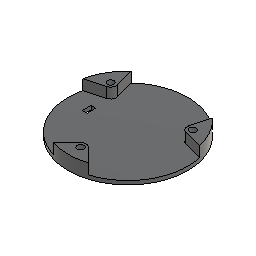
RGB_ChristmasLight_Base_Enclosure_Bottom_v1 (Autodesk Fusion 360 design; units mm, degrees)
Autodesk Fusion 360 part; units mm, degrees
(part 1 of 2)
sketch "Sketch1" plane through (0, 0, 0) normal (0, 0, 1) x (1, 0, 0)
  circle A0 centre (0, 0) radius 31.5
  circle A1 centre (0, 0) radius 30 construction
  circle A2 centre (0, 0) radius 25 construction
  circle A3 centre (0, -25) radius 1.75
  circle A4 centre (21.6506, 12.5) radius 1.75
  circle A5 centre (-21.6506, 12.5) radius 1.75
  line L0 (-30, 0) -> (-20.5, 0) construction
  line L1 (-20.5, 0) -> (-19.25, 0) construction
  line L2 (-19.25, 0) -> (-19.25, 2.25) construction
  line L3 (-19.25, 2.25) -> (-20.5, 2.25) construction
  line L4 (-20.5, 2.25) -> (-20.5, 0) construction
  line L5 (-19.25, 2.25) -> (-21.75, 2.25)
  line L6 (-21.75, 2.25) -> (-21.75, -2.25)
  line L7 (-21.75, -2.25) -> (-19.25, -2.25)
  line L8 (-19.25, -2.25) -> (-19.25, 2.25)
  dimension "d1_1" = 63
  dimension "d84" = 60
  dimension "d85" = -5
  dimension "d86" = 3.5
  dimension "d88" = 360
  dimension "d89" = 9.5
  dimension "d90" = 1.25
  dimension "d91" = 2.25
  dimension "d92" = 2.5
  dimension "d93" = 4.5
  constraint coincident A0.centre A1.centre
  constraint coincident A2 A3.centre
  constraint coincident A1 L0.start
  constraint horizontal L0
  constraint horizontal L1
  constraint vertical L2
  constraint horizontal L3
  constraint vertical L4
  constraint horizontal L5
  constraint vertical L6
  constraint horizontal L7
  constraint vertical L8
  measures "d1_1" diameter of A0
  measures "d84" diameter of A1
  measures "d86" diameter of A3
  measures "d89" distance of L0.start L0.end
  measures "d90" distance of L0.end L1.end
  measures "d91" distance of L0.end L3.end
  measures "d92" distance of L2.end L5.end
  measures "d93" distance of L2.end L7.end
extrude "Extrude1" add sketch "Sketch1" along normal blind 2 contours A0 | A3 | A4 | A5 | L5 L6 L7 L8
extrude "Extrude5" cut sketch "Sketch1" along normal blind 2 contours A3 | A4 | A5 | L5 L6 L7 L8
sketch "Sketch3" plane through (0, 0, 2) normal (0, 0, 1) x (-1, 0, 0)
  line L0 (19.25, 2.25) -> (21.75, 2.25)
  line L1 (21.75, 2.25) -> (21.75, -2.25)
  line L2 (21.75, -2.25) -> (19.25, -2.25)
  line L3 (19.25, -2.25) -> (19.25, 2.25)
  circle A0 centre (0, 25) radius 1.75
  circle A1 centre (21.6506, -12.5) radius 1.75
  circle A2 centre (-21.6506, -12.5) radius 1.75
  circle A3 centre (0, 0) radius 31.5
  arc A4 (2.1213, 22.8787) -> (0, 22) centre (0, 25) cw
  arc A5 (0, 22) -> (-2.1213, 22.8787) centre (0, 25) cw
  line L4 (-2.1213, 22.8787) -> (-9.3294, 30.0867)
  line L5 (2.1213, 22.8787) -> (9.3294, 30.0867)
  line L6 (-20.8742, -9.6022) -> (-30.7206, -6.9639)
  arc A6 (-20.8742, -9.6022) -> (-19.0526, -11) centre (-21.6506, -12.5) cw
  arc A7 (-19.0526, -11) -> (-18.7529, -13.2765) centre (-21.6506, -12.5) cw
  line L7 (-18.7529, -13.2765) -> (-21.3912, -23.1229)
  line L8 (18.7529, -13.2765) -> (21.3912, -23.1229)
  arc A8 (18.7529, -13.2765) -> (19.0526, -11) centre (21.6506, -12.5) cw
  arc A9 (19.0526, -11) -> (20.8742, -9.6022) centre (21.6506, -12.5) cw
  line L9 (20.8742, -9.6022) -> (30.7206, -6.9639)
  dimension "d108" = 360
extrude "Extrude6" add sketch "Sketch3" along normal blind 5.45 contours A3 A4 A5 L4 L5 | A3 L8 A8 A9 L9 | A3 L6 A6 A7 L7
sketch "Sketch4" plane through (0, 0, 0) normal (0, 0, -1) x (1, 0, 0)
  line L0 (-21.75, 2.25) -> (-19.25, 2.25)
  line L1 (-19.25, 2.25) -> (-19.25, -2.25)
  line L2 (-19.25, -2.25) -> (-21.75, -2.25)
  line L3 (-21.75, -2.25) -> (-21.75, 2.25)
  circle A0 centre (0, 25) radius 1.75
  circle A1 centre (-21.6506, -12.5) radius 1.75
  circle A2 centre (21.6506, -12.5) radius 1.75
  circle A3 centre (0, 0) radius 31.5
  spline S0 degree 3 poles (-1.0856, -16.0234) (-1.0936, -16.0234) (-1.2047, -15.8091) (-1.3357, -15.5472) knots 0 0 0 0 1 1 1 1
  spline S1 degree 3 poles (-1.3357, -15.5472) (-1.4666, -15.2852) (-1.5738, -15.0551) (-1.5738, -15.0312) knots 0 0 0 0 1 1 1 1
  spline S2 degree 3 poles (-1.5738, -15.0312) (-1.5738, -14.9916) (-1.1491, -15.0074) (-0.6729, -15.067) knots 0 0 0 0 1 1 1 1
  line L4 (-0.6729, -15.067) -> (-0.4626, -15.0908)
  line L5 (-0.4626, -15.0908) -> (-0.7721, -15.5551)
  spline S3 degree 3 poles (-0.7721, -15.5551) (-0.9388, -15.8131) (-1.0817, -16.0234) (-1.0856, -16.0234) knots 0 0 0 0 1 1 1 1
  spline S4 degree 3 poles (15.4005, 7.3843) (15.3728, 7.3684) (14.8806, 7.0787) (14.3012, 6.7413) knots -1 -1 -1 -1 0 0 0 0
  spline S5 degree 3 poles (14.7139, 8.682) (15.2219, 7.8049) (15.4323, 7.4041) (15.4005, 7.3843) knots -1 -1 -1 -1 0 0 0 0
  spline S6 degree 3 poles (13.948, 9.9838) (13.9639, 9.9679) (14.3091, 9.3805) (14.7139, 8.682) knots -1 -1 -1 -1 0 0 0 0
  spline S7 degree 3 poles (13.6583, 9.8608) (13.8011, 9.9441) (13.9321, 9.9997) (13.948, 9.9838) knots -1 -1 -1 -1 0 0 0 0
  line L6 (13.3963, 9.7099) -> (13.6583, 9.8608)
  line L7 (14.3726, 8.0272) -> (13.3963, 9.7099)
  line L8 (14.2496, 7.9518) -> (14.3726, 8.0272)
  spline S8 degree 3 poles (13.4876, 7.5113) (13.8369, 7.7137) (14.1782, 7.9121) (14.2496, 7.9518) knots -1 -1 -1 -1 0 0 0 0
  spline S9 degree 3 poles (12.7653, 7.0906) (12.8129, 7.1223) (13.1384, 7.3089) (13.4876, 7.5113) knots -1 -1 -1 -1 0 0 0 0
  spline S10 degree 3 poles (12.9439, 6.5786) (12.6819, 7.035) (12.6819, 7.039) (12.7653, 7.0906) knots -1 -1 -1 -1 0 0 0 0
  spline S11 degree 3 poles (13.2296, 6.1262) (13.2177, 6.1222) (13.0907, 6.3286) (12.9439, 6.5786) knots -1 -1 -1 -1 0 0 0 0
  spline S12 degree 3 poles (14.3012, 6.7413) (13.7218, 6.404) (13.2415, 6.1262) (13.2296, 6.1262) knots -1 -1 -1 -1 0 0 0 0
  spline S13 degree 3 poles (-13.8214, 4.5545) (-13.8293, 3.7092) (-14.2262, 2.8599) (-14.7104, 2.6535) knots -1 -1 -1 -1 0 0 0 0
  spline S14 degree 3 poles (-13.9325, 5.1618) (-13.8253, 4.9673) (-13.8174, 4.9236) (-13.8214, 4.5545) knots -1 -1 -1 -1 0 0 0 0
  spline S15 degree 3 poles (-14.7104, 5.6063) (-14.4286, 5.6817) (-14.127, 5.507) (-13.9325, 5.1618) knots -1 -1 -1 -1 0 0 0 0
  spline S16 degree 3 poles (-15.4843, 4.4156) (-15.2025, 5.2094) (-14.9921, 5.5308) (-14.7104, 5.6063) knots -1 -1 -1 -1 0 0 0 0
  spline S17 degree 3 poles (-15.8454, 4.0386) (-15.7383, 3.7886) (-15.6867, 3.8441) (-15.4843, 4.4156) knots -1 -1 -1 -1 0 0 0 0
  spline S18 degree 3 poles (-15.6827, 4.6538) (-15.8613, 4.4672) (-15.9248, 4.2291) (-15.8454, 4.0386) knots -1 -1 -1 -1 0 0 0 0
  spline S19 degree 3 poles (-15.5279, 4.8919) (-15.5438, 4.8363) (-15.6113, 4.7292) (-15.6827, 4.6538) knots -1 -1 -1 -1 0 0 0 0
  spline S20 degree 3 poles (-15.389, 5.4158) (-15.4525, 5.1816) (-15.516, 4.9474) (-15.5279, 4.8919) knots -1 -1 -1 -1 0 0 0 0
  line L9 (-15.2739, 5.8444) -> (-15.389, 5.4158)
  line L10 (-15.4366, 5.8206) -> (-15.2739, 5.8444)
  spline S21 degree 3 poles (-16.54, 4.4275) (-16.3415, 5.2848) (-15.9843, 5.7333) (-15.4366, 5.8206) knots -1 -1 -1 -1 0 0 0 0
  spline S22 degree 3 poles (-16.2145, 2.9115) (-16.5955, 3.1853) (-16.7066, 3.7013) (-16.54, 4.4275) knots -1 -1 -1 -1 0 0 0 0
  spline S23 degree 3 poles (-14.9088, 4.0465) (-15.3255, 2.8519) (-15.6946, 2.5305) (-16.2145, 2.9115) knots -1 -1 -1 -1 0 0 0 0
  spline S24 degree 3 poles (-14.6111, 4.4315) (-14.6985, 4.5466) (-14.762, 4.4633) (-14.9088, 4.0465) knots -1 -1 -1 -1 0 0 0 0
  spline S25 degree 3 poles (-14.762, 3.7171) (-14.5715, 3.864) (-14.4841, 4.2648) (-14.6111, 4.4315) knots -1 -1 -1 -1 0 0 0 0
  spline S26 degree 3 poles (-14.9882, 3.1853) (-14.889, 3.5425) (-14.8413, 3.6576) (-14.762, 3.7171) knots -1 -1 -1 -1 0 0 0 0
  spline S27 degree 3 poles (-15.1311, 2.6575) (-15.1191, 2.6972) (-15.0556, 2.9353) (-14.9882, 3.1853) knots -1 -1 -1 -1 0 0 0 0
  spline S28 degree 3 poles (-15.0001, 2.59) (-15.1271, 2.59) (-15.1469, 2.6019) (-15.1311, 2.6575) knots -1 -1 -1 -1 0 0 0 0
  spline S29 degree 3 poles (-14.7104, 2.6535) (-14.7858, 2.6218) (-14.9167, 2.594) (-15.0001, 2.59) knots -1 -1 -1 -1 0 0 0 0
  spline S30 degree 3 poles (16.7856, 3.1893) (16.7658, 3.1814) (16.2181, 3.0266) (15.5752, 2.848) knots -1 -1 -1 -1 0 0 0 0
  spline S31 degree 3 poles (15.9998, 6.1857) (16.0474, 6.1381) (16.8174, 3.2012) (16.7856, 3.1893) knots -1 -1 -1 -1 0 0 0 0
  spline S32 degree 3 poles (15.4244, 6.0269) (15.4482, 6.0508) (15.9839, 6.1976) (15.9998, 6.1857) knots -1 -1 -1 -1 0 0 0 0
  spline S33 degree 3 poles (15.6704, 5.0506) (15.5275, 5.5824) (15.4164, 6.019) (15.4244, 6.0269) knots -1 -1 -1 -1 0 0 0 0
  spline S34 degree 3 poles (15.9165, 4.0743) (15.9284, 4.0823) (15.8173, 4.5228) (15.6704, 5.0506) knots -1 -1 -1 -1 0 0 0 0
  spline S35 degree 3 poles (15.718, 3.9989) (15.8173, 4.0267) (15.9046, 4.0624) (15.9165, 4.0743) knots -1 -1 -1 -1 0 0 0 0
  line L11 (15.5355, 3.9434) -> (15.718, 3.9989)
  line L12 (15.4759, 4.1497) -> (15.5355, 3.9434)
  spline S36 degree 3 poles (15.2696, 4.8919) (15.3529, 4.5982) (15.4442, 4.2648) (15.4759, 4.1497) knots -1 -1 -1 -1 0 0 0 0
  spline S37 degree 3 poles (15.0949, 5.4594) (15.1108, 5.4435) (15.1902, 5.1856) (15.2696, 4.8919) knots -1 -1 -1 -1 0 0 0 0
  spline S38 degree 3 poles (14.6862, 5.3681) (14.7497, 5.4197) (15.0672, 5.4912) (15.0949, 5.4594) knots -1 -1 -1 -1 0 0 0 0
  spline S39 degree 3 poles (14.8568, 4.5942) (14.7457, 5.003) (14.6663, 5.3523) (14.6862, 5.3681) knots -1 -1 -1 -1 0 0 0 0
  spline S40 degree 3 poles (15.0434, 3.8322) (15.0513, 3.8441) (14.9679, 4.1854) (14.8568, 4.5942) knots -1 -1 -1 -1 0 0 0 0
  spline S41 degree 3 poles (14.8409, 3.7608) (14.9402, 3.7886) (15.0314, 3.8243) (15.0434, 3.8322) knots -1 -1 -1 -1 0 0 0 0
  spline S42 degree 3 poles (14.6385, 3.7529) (14.6504, 3.7132) (14.6981, 3.7171) (14.8409, 3.7608) knots -1 -1 -1 -1 0 0 0 0
  spline S43 degree 3 poles (14.3964, 4.6339) (14.5195, 4.1735) (14.6306, 3.7806) (14.6385, 3.7529) knots -1 -1 -1 -1 0 0 0 0
  spline S44 degree 3 poles (14.1424, 5.4991) (14.1583, 5.4832) (14.2734, 5.0903) (14.3964, 4.6339) knots -1 -1 -1 -1 0 0 0 0
  spline S45 degree 3 poles (13.5709, 5.3245) (13.567, 5.388) (14.0988, 5.5507) (14.1424, 5.4991) knots -1 -1 -1 -1 0 0 0 0
  spline S46 degree 3 poles (14.2655, 2.7765) (14.1147, 3.3044) (13.5749, 5.2689) (13.5709, 5.3245) knots -1 -1 -1 -1 0 0 0 0
  spline S47 degree 3 poles (14.3726, 2.5146) (14.3568, 2.5106) (14.3091, 2.6297) (14.2655, 2.7765) knots -1 -1 -1 -1 0 0 0 0
  spline S48 degree 3 poles (15.5752, 2.848) (14.9283, 2.6654) (14.3885, 2.5186) (14.3726, 2.5146) knots -1 -1 -1 -1 0 0 0 0
  spline S49 degree 3 poles (8.3917, 2.8242) (8.4513, 2.6337) (8.3838, 2.4313) (8.225, 2.2924) knots -1 -1 -1 -1 0 0 0 0
  spline S50 degree 3 poles (7.9353, 3.1774) (8.1893, 3.1575) (8.3243, 3.0504) (8.3917, 2.8242) knots -1 -1 -1 -1 0 0 0 0
  spline S51 degree 3 poles (7.5702, 3.0544) (7.7131, 3.1853) (7.7369, 3.1933) (7.9353, 3.1774) knots -1 -1 -1 -1 0 0 0 0
  spline S52 degree 3 poles (7.4154, 2.6892) (7.4154, 2.8996) (7.4273, 2.9234) (7.5702, 3.0544) knots -1 -1 -1 -1 0 0 0 0
  spline S53 degree 3 poles (7.5623, 2.3281) (7.4273, 2.4551) (7.4154, 2.4789) (7.4154, 2.6892) knots -1 -1 -1 -1 0 0 0 0
  spline S54 degree 3 poles (7.9075, 2.1931) (7.7409, 2.1931) (7.6893, 2.213) (7.5623, 2.3281) knots -1 -1 -1 -1 0 0 0 0
  spline S55 degree 3 poles (8.225, 2.2924) (8.1298, 2.2169) (8.0584, 2.1931) (7.9075, 2.1931) knots -1 -1 -1 -1 0 0 0 0
  spline S56 degree 3 poles (-8.2016, 3.0663) (-7.7016, 3.0663) (-7.5071, 2.4709) (-7.9079, 2.1574) knots -1 -1 -1 -1 0 0 0 0
  spline S57 degree 3 poles (-8.658, 2.7884) (-8.5628, 2.975) (-8.412, 3.0663) (-8.2016, 3.0663) knots -1 -1 -1 -1 0 0 0 0
  spline S58 degree 3 poles (-8.2016, 2.0741) (-8.5826, 2.0741) (-8.8287, 2.4551) (-8.658, 2.7884) knots -1 -1 -1 -1 0 0 0 0
  spline S59 degree 3 poles (-7.9079, 2.1574) (-7.9833, 2.0979) (-8.0706, 2.0741) (-8.2016, 2.0741) knots -1 -1 -1 -1 0 0 0 0
  spline S60 degree 3 poles (6.963, -0.1326) (7.0622, -0.3548) (7.0146, -0.5691) (6.836, -0.7199) knots -1 -1 -1 -1 0 0 0 0
  spline S61 degree 3 poles (6.0065, -0.327) (6.0065, 0.2167) (6.7447, 0.3635) (6.963, -0.1326) knots -1 -1 -1 -1 0 0 0 0
  spline S62 degree 3 poles (6.5383, -0.8231) (6.2089, -0.8231) (6.0065, -0.6366) (6.0065, -0.327) knots -1 -1 -1 -1 0 0 0 0
  spline S63 degree 3 poles (6.836, -0.7199) (6.7447, -0.7993) (6.6693, -0.8231) (6.5383, -0.8231) knots -1 -1 -1 -1 0 0 0 0
  spline S64 degree 3 poles (10.134, 0.7287) (10.134, 0.5818) (10.1102, 0.5342) (9.9792, 0.4032) knots -1 -1 -1 -1 0 0 0 0
  spline S65 degree 3 poles (9.3045, 1.1374) (9.6498, 1.4311) (10.134, 1.193) (10.134, 0.7287) knots -1 -1 -1 -1 0 0 0 0
  spline S66 degree 3 poles (9.2172, 0.4509) (9.0744, 0.7168) (9.1061, 0.9747) (9.3045, 1.1374) knots -1 -1 -1 -1 0 0 0 0
  spline S67 degree 3 poles (9.6617, 0.2484) (9.4673, 0.2484) (9.2807, 0.3358) (9.2172, 0.4509) knots -1 -1 -1 -1 0 0 0 0
  spline S68 degree 3 poles (9.9792, 0.4032) (9.8522, 0.2723) (9.8006, 0.2484) (9.6617, 0.2484) knots -1 -1 -1 -1 0 0 0 0
  spline S69 degree 3 poles (-5.9394, 0.4469) (-5.9394, 0.1849) (-6.0863, -0.0214) (-6.3165, -0.081) knots -1 -1 -1 -1 0 0 0 0
  spline S70 degree 3 poles (-6.3641, 0.9112) (-6.1299, 0.8795) (-5.9394, 0.6731) (-5.9394, 0.4469) knots -1 -1 -1 -1 0 0 0 0
  spline S71 degree 3 poles (-6.9475, 0.4866) (-6.8959, 0.7842) (-6.6697, 0.9509) (-6.3641, 0.9112) knots -1 -1 -1 -1 0 0 0 0
  spline S72 degree 3 poles (-6.3165, -0.081) (-6.6419, -0.1643) (-7.007, 0.1611) (-6.9475, 0.4866) knots -1 -1 -1 -1 0 0 0 0
  spline S73 degree 3 poles (8.5187, -10.4156) (6.2645, -12.2134) (3.6332, -13.2374) (0.8273, -13.4041) knots -1 -1 -1 -1 0 0 0 0
  spline S74 degree 3 poles (10.5071, -8.4233) (10.0705, -8.971) (9.0545, -9.987) (8.5187, -10.4156) knots -1 -1 -1 -1 0 0 0 0
  spline S75 degree 3 poles (13.3249, -2.0852) (12.9677, -4.3632) (11.9954, -6.558) (10.5071, -8.4233) knots -1 -1 -1 -1 0 0 0 0
  line L13 (13.3765, -1.7359) -> (13.3249, -2.0852)
  line L14 (11.9676, -1.7359) -> (13.3765, -1.7359)
  line L15 (11.7255, -2.1487) -> (11.9676, -1.7359)
  spline S76 degree 3 poles (11.4358, -2.5773) (11.4635, -2.5694) (11.5945, -2.3749) (11.7255, -2.1487) knots -1 -1 -1 -1 0 0 0 0
  spline S77 degree 3 poles (10.1856, -2.5932) (10.8444, -2.5932) (11.408, -2.5892) (11.4358, -2.5773) knots -1 -1 -1 -1 0 0 0 0
  line L16 (8.991, -2.5892) -> (10.1856, -2.5932)
  line L17 (8.9474, -2.7361) -> (8.991, -2.5892)
  spline S78 degree 3 poles (8.5187, -3.1686) (8.6854, -3.1051) (8.8997, -2.8869) (8.9474, -2.7361) knots -1 -1 -1 -1 0 0 0 0
  spline S79 degree 3 poles (7.979, -3.1488) (8.1298, -3.2123) (8.3798, -3.2202) (8.5187, -3.1686) knots -1 -1 -1 -1 0 0 0 0
  spline S80 degree 3 poles (7.5146, -2.4701) (7.5146, -2.7083) (7.7528, -3.0575) (7.979, -3.1488) knots -1 -1 -1 -1 0 0 0 0
  spline S81 degree 3 poles (7.717, -1.9939) (7.6139, -2.113) (7.5146, -2.3471) (7.5146, -2.4701) knots -1 -1 -1 -1 0 0 0 0
  spline S82 degree 3 poles (8.9275, -2.1884) (8.7291, -1.7002) (8.0663, -1.597) (7.717, -1.9939) knots -1 -1 -1 -1 0 0 0 0
  line L18 (9.0029, -2.3709) -> (8.9275, -2.1884)
  line L19 (11.3445, -2.3709) -> (9.0029, -2.3709)
  line L20 (11.5826, -1.9621) -> (11.3445, -2.3709)
  line L21 (11.8207, -1.5573) -> (11.5826, -1.9621)
  line L22 (12.6026, -1.5454) -> (11.8207, -1.5573)
  spline S83 degree 3 poles (13.4003, -1.4819) (13.3844, -1.5256) (13.2019, -1.5375) (12.6026, -1.5454) knots -1 -1 -1 -1 0 0 0 0
  spline S84 degree 3 poles (13.4479, -1.0295) (13.432, -1.2478) (13.4122, -1.4541) (13.4003, -1.4819) knots -1 -1 -1 -1 0 0 0 0
  spline S85 degree 3 poles (13.4241, -0.6207) (13.4678, -0.6247) (13.4717, -0.7001) (13.4479, -1.0295) knots -1 -1 -1 -1 0 0 0 0
  spline S86 degree 3 poles (12.0985, -0.6128) (12.797, -0.6128) (13.3924, -0.6167) (13.4241, -0.6207) knots -1 -1 -1 -1 0 0 0 0
  spline S87 degree 3 poles (10.7809, -0.6644) (10.8246, -0.6128) (11.0151, -0.6048) (12.0985, -0.6128) knots -1 -1 -1 -1 0 0 0 0
  spline S88 degree 3 poles (10.5626, -0.9819) (10.6539, -0.839) (10.7531, -0.6961) (10.7809, -0.6644) knots -1 -1 -1 -1 0 0 0 0
  line L23 (10.392, -1.2398) -> (10.5626, -0.9819)
  line L24 (9.4554, -1.2517) -> (10.392, -1.2398)
  spline S89 degree 3 poles (8.225, -0.7874) (8.5068, -1.3113) (8.3759, -1.2636) (9.4554, -1.2517) knots -1 -1 -1 -1 0 0 0 0
  line L25 (8.0425, -0.4461) -> (8.225, -0.7874)
  line L26 (7.2567, -0.4223) -> (8.0425, -0.4461)
  line L27 (7.1654, -0.6247) -> (7.2567, -0.4223)
  spline S90 degree 3 poles (5.9787, -0.8112) (6.3439, -1.1962) (6.9471, -1.1009) (7.1654, -0.6247) knots -1 -1 -1 -1 0 0 0 0
  spline S91 degree 3 poles (6.0938, 0.2723) (5.7168, 0.0143) (5.6652, -0.4818) (5.9787, -0.8112) knots -1 -1 -1 -1 0 0 0 0
  spline S92 degree 3 poles (6.5026, 0.3874) (6.2962, 0.3874) (6.2327, 0.3675) (6.0938, 0.2723) knots -1 -1 -1 -1 0 0 0 0
  spline S93 degree 3 poles (7.1694, -0.0333) (7.0503, 0.2484) (6.828, 0.3874) (6.5026, 0.3874) knots -1 -1 -1 -1 0 0 0 0
  line L28 (7.2527, -0.2278) -> (7.1694, -0.0333)
  line L29 (8.1734, -0.2278) -> (7.2527, -0.2278)
  line L30 (8.3878, -0.6247) -> (8.1734, -0.2278)
  line L31 (8.5981, -1.0216) -> (8.3878, -0.6247)
  line L32 (10.2848, -1.0216) -> (8.5981, -1.0216)
  line L33 (10.6896, -0.3866) -> (10.2848, -1.0216)
  line L34 (12.0747, -0.3866) -> (10.6896, -0.3866)
  spline S94 degree 3 poles (13.4836, -0.3231) (13.4638, -0.3786) (13.3011, -0.3866) (12.0747, -0.3866) knots -1 -1 -1 -1 0 0 0 0
  spline S95 degree 3 poles (13.4836, 0.435) (13.5154, 0.1691) (13.5154, -0.2437) (13.4836, -0.3231) knots -1 -1 -1 -1 0 0 0 0
  line L35 (13.4559, 0.6453) -> (13.4836, 0.435)
  line L36 (10.3721, 0.6453) -> (13.4559, 0.6453)
  line L37 (10.3086, 0.4866) -> (10.3721, 0.6453)
  spline S96 degree 3 poles (9.5268, 0.0302) (9.8165, -0.0294) (10.1856, 0.1849) (10.3086, 0.4866) knots -1 -1 -1 -1 0 0 0 0
  spline S97 degree 3 poles (9.2053, 1.3438) (8.6854, 0.9469) (8.8759, 0.1691) (9.5268, 0.0302) knots -1 -1 -1 -1 0 0 0 0
  spline S98 degree 3 poles (9.9673, 1.4034) (9.7371, 1.5224) (9.4038, 1.4946) (9.2053, 1.3438) knots -1 -1 -1 -1 0 0 0 0
  spline S99 degree 3 poles (10.3324, 0.9549) (10.3324, 1.0779) (10.138, 1.316) (9.9673, 1.4034) knots -1 -1 -1 -1 0 0 0 0
  spline S100 degree 3 poles (10.3999, 0.8795) (10.3642, 0.8834) (10.3324, 0.9152) (10.3324, 0.9549) knots -1 -1 -1 -1 0 0 0 0
  spline S101 degree 3 poles (13.3844, 0.8795) (13.2654, 0.8755) (10.4952, 0.8755) (10.3999, 0.8795) knots -1 -1 -1 -1 0 0 0 0
  spline S102 degree 3 poles (13.4519, 1.1017) (13.4757, 0.8914) (13.4717, 0.8834) (13.3844, 0.8795) knots -1 -1 -1 -1 0 0 0 0
  spline S103 degree 3 poles (13.4043, 1.5383) (13.4162, 1.4192) (13.44, 1.2208) (13.4519, 1.1017) knots -1 -1 -1 -1 0 0 0 0
  line L38 (13.3804, 1.7566) -> (13.4043, 1.5383)
  line L39 (11.9239, 1.7566) -> (13.3804, 1.7566)
  spline S104 degree 3 poles (10.4277, 1.7883) (10.4515, 1.7724) (11.1262, 1.7566) (11.9239, 1.7566) knots -1 -1 -1 -1 0 0 0 0
  spline S105 degree 3 poles (10.1142, 2.2011) (10.265, 1.9907) (10.4039, 1.8042) (10.4277, 1.7883) knots -1 -1 -1 -1 0 0 0 0
  line L40 (9.8443, 2.59) -> (10.1142, 2.2011)
  line L41 (8.6338, 2.59) -> (9.8443, 2.59)
  line L42 (8.606, 2.4789) -> (8.6338, 2.59)
  spline S106 degree 3 poles (8.229, 2.0344) (8.4036, 2.1217) (8.5664, 2.3162) (8.606, 2.4789) knots -1 -1 -1 -1 0 0 0 0
  spline S107 degree 3 poles (7.217, 2.4392) (7.3916, 2.0264) (7.852, 1.8399) (8.229, 2.0344) knots -1 -1 -1 -1 0 0 0 0
  spline S108 degree 3 poles (7.2329, 2.967) (7.1416, 2.7726) (7.1376, 2.6337) (7.217, 2.4392) knots -1 -1 -1 -1 0 0 0 0
  spline S109 degree 3 poles (8.5624, 2.9829) (8.3084, 3.5624) (7.4988, 3.5504) (7.2329, 2.967) knots -1 -1 -1 -1 0 0 0 0
  line L43 (8.6457, 2.7884) -> (8.5624, 2.9829)
  line L44 (9.9713, 2.7884) -> (8.6457, 2.7884)
  line L45 (10.2412, 2.3916) -> (9.9713, 2.7884)
  line L46 (10.511, 1.9987) -> (10.2412, 2.3916)
  line L47 (11.9279, 1.9947) -> (10.511, 1.9987)
  spline S110 degree 3 poles (13.3487, 2.0304) (13.3487, 2.0106) (12.801, 1.9947) (11.9279, 1.9947) knots -1 -1 -1 -1 0 0 0 0
  spline S111 degree 3 poles (13.2654, 2.4987) (13.313, 2.2646) (13.3487, 2.0542) (13.3487, 2.0304) knots -1 -1 -1 -1 0 0 0 0
  spline S112 degree 3 poles (9.376, 9.7139) (11.4278, 7.7216) (12.7296, 5.3046) (13.2654, 2.4987) knots -1 -1 -1 -1 0 0 0 0
  spline S113 degree 3 poles (-2.2763, 13.3017) (2.0378, 14.024) (6.2843, 12.7143) (9.376, 9.7139) knots -1 -1 -1 -1 0 0 0 0
  spline S114 degree 3 poles (-8.0905, 10.7775) (-6.3958, 12.0634) (-4.3321, 12.9603) (-2.2763, 13.3017) knots -1 -1 -1 -1 0 0 0 0
  spline S115 degree 3 poles (-13.1784, 2.6694) (-12.5474, 5.8841) (-10.7376, 8.7693) (-8.0905, 10.7775) knots -1 -1 -1 -1 0 0 0 0
  spline S116 degree 3 poles (-13.2975, 2.0026) (-13.2856, 2.0979) (-13.23, 2.3955) (-13.1784, 2.6694) knots -1 -1 -1 -1 0 0 0 0
  line L48 (-13.3213, 1.8359) -> (-13.2975, 2.0026)
  line L49 (-11.8965, 1.8359) -> (-13.3213, 1.8359)
  line L50 (-11.6544, 2.2527) -> (-11.8965, 1.8359)
  line L51 (-11.4084, 2.6694) -> (-11.6544, 2.2527)
  line L52 (-8.9239, 2.6694) -> (-11.4084, 2.6694)
  line L53 (-8.8961, 2.7924) -> (-8.9239, 2.6694)
  spline S117 degree 3 poles (-8.1619, 3.3044) (-8.4755, 3.3044) (-8.8366, 3.0543) (-8.8961, 2.7924) knots -1 -1 -1 -1 0 0 0 0
  spline S118 degree 3 poles (-7.4912, 2.7289) (-7.5746, 3.0385) (-7.8801, 3.3004) (-8.1619, 3.3044) knots -1 -1 -1 -1 0 0 0 0
  spline S119 degree 3 poles (-8.5072, 1.9074) (-7.9794, 1.6415) (-7.3404, 2.1574) (-7.4912, 2.7289) knots -1 -1 -1 -1 0 0 0 0
  spline S120 degree 3 poles (-8.9041, 2.3558) (-8.8723, 2.2011) (-8.7017, 2.0066) (-8.5072, 1.9074) knots -1 -1 -1 -1 0 0 0 0
  line L54 (-8.9279, 2.4709) -> (-8.9041, 2.3558)
  line L55 (-11.2774, 2.4709) -> (-8.9279, 2.4709)
  line L56 (-11.4719, 2.1296) -> (-11.2774, 2.4709)
  spline S121 degree 3 poles (-12.5553, 1.6097) (-11.6901, 1.6177) (-11.7933, 1.57) (-11.4719, 2.1296) knots -1 -1 -1 -1 0 0 0 0
  spline S122 degree 3 poles (-13.3292, 1.6018) (-13.3134, 1.6018) (-12.9641, 1.6097) (-12.5553, 1.6097) knots -1 -1 -1 -1 0 0 0 0
  spline S123 degree 3 poles (-13.3769, 1.2486) (-13.365, 1.443) (-13.3411, 1.5978) (-13.3292, 1.6018) knots -1 -1 -1 -1 0 0 0 0
  spline S124 degree 3 poles (-13.4205, 0.7922) (-13.4126, 0.8557) (-13.3927, 1.0581) (-13.3769, 1.2486) knots -1 -1 -1 -1 0 0 0 0
  line L57 (-13.4404, 0.685) -> (-13.4205, 0.7922)
  line L58 (-10.7535, 0.685) -> (-13.4404, 0.685)
  line L59 (-10.5392, 1.0104) -> (-10.7535, 0.685)
  line L60 (-10.3249, 1.3398) -> (-10.5392, 1.0104)
  line L61 (-9.3803, 1.3518) -> (-10.3249, 1.3398)
  line L62 (-8.4397, 1.3597) -> (-9.3803, 1.3518)
  line L63 (-8.3604, 1.2327) -> (-8.4397, 1.3597)
  spline S125 degree 3 poles (-8.1302, 0.816) (-8.2135, 0.9708) (-8.3167, 1.1613) (-8.3604, 1.2327) knots -1 -1 -1 -1 0 0 0 0
  line L64 (-7.9833, 0.5263) -> (-8.1302, 0.816)
  line L65 (-7.1777, 0.5263) -> (-7.9833, 0.5263)
  line L66 (-7.1301, 0.6612) -> (-7.1777, 0.5263)
  spline S126 degree 3 poles (-6.6657, 1.1057) (-6.8205, 1.07) (-7.0785, 0.8239) (-7.1301, 0.6612) knots -1 -1 -1 -1 0 0 0 0
  spline S127 degree 3 poles (-6.499, 1.1454) (-6.5308, 1.1374) (-6.6022, 1.1176) (-6.6657, 1.1057) knots -1 -1 -1 -1 0 0 0 0
  spline S128 degree 3 poles (-6.2807, 1.1176) (-6.372, 1.1414) (-6.4712, 1.1533) (-6.499, 1.1454) knots -1 -1 -1 -1 0 0 0 0
  spline S129 degree 3 poles (-5.8362, 0.0103) (-5.5545, 0.4389) (-5.7727, 0.9827) (-6.2807, 1.1176) knots -1 -1 -1 -1 0 0 0 0
  spline S130 degree 3 poles (-6.7451, -0.2516) (-6.4236, -0.3866) (-6.0228, -0.2715) (-5.8362, 0.0103) knots -1 -1 -1 -1 0 0 0 0
  spline S131 degree 3 poles (-7.138, 0.177) (-7.0824, 0.0143) (-6.8919, -0.1921) (-6.7451, -0.2516) knots -1 -1 -1 -1 0 0 0 0
  line L67 (-7.1777, 0.2842) -> (-7.138, 0.177)
  line L68 (-7.6381, 0.2961) -> (-7.1777, 0.2842)
  line L69 (-8.1024, 0.308) -> (-7.6381, 0.2961)
  line L70 (-8.3207, 0.7128) -> (-8.1024, 0.308)
  line L71 (-8.539, 1.1216) -> (-8.3207, 0.7128)
  line L72 (-10.2098, 1.1216) -> (-8.539, 1.1216)
  line L73 (-10.4162, 0.8041) -> (-10.2098, 1.1216)
  line L74 (-10.6186, 0.4866) -> (-10.4162, 0.8041)
  line L75 (-13.4404, 0.4866) -> (-10.6186, 0.4866)
  line L76 (-13.4404, -0.5453) -> (-13.4404, 0.4866)
  line L77 (-10.309, -0.5453) -> (-13.4404, -0.5453)
  line L78 (-10.2336, -0.3707) -> (-10.309, -0.5453)
  spline S132 degree 3 poles (-10.0034, -0.0849) (-10.0868, -0.1484) (-10.19, -0.2754) (-10.2336, -0.3707) knots -1 -1 -1 -1 0 0 0 0
  spline S133 degree 3 poles (-9.5708, 0.0302) (-9.8248, 0.0302) (-9.8725, 0.0183) (-10.0034, -0.0849) knots -1 -1 -1 -1 0 0 0 0
  spline S134 degree 3 poles (-9.1422, -0.081) (-9.2692, 0.0183) (-9.3208, 0.0302) (-9.5708, 0.0302) knots -1 -1 -1 -1 0 0 0 0
  spline S135 degree 3 poles (-8.9835, -1.093) (-8.7414, -0.7914) (-8.8128, -0.331) (-9.1422, -0.081) knots -1 -1 -1 -1 0 0 0 0
  spline S136 degree 3 poles (-9.5708, -1.3946) (-9.3327, -1.3946) (-9.1581, -1.3073) (-8.9835, -1.093) knots -1 -1 -1 -1 0 0 0 0
  spline S137 degree 3 poles (-10.2455, -0.9303) (-10.1185, -1.2319) (-9.8883, -1.3867) (-9.5708, -1.3946) knots -1 -1 -1 -1 0 0 0 0
  line L79 (-10.3051, -0.7834) -> (-10.2455, -0.9303)
  line L80 (-13.4126, -0.7834) -> (-10.3051, -0.7834)
  line L81 (-13.3848, -1.1525) -> (-13.4126, -0.7834)
  spline S138 degree 3 poles (-13.3332, -1.605) (-13.3491, -1.5573) (-13.3689, -1.351) (-13.3848, -1.1525) knots -1 -1 -1 -1 0 0 0 0
  line L82 (-13.3134, -1.6962) -> (-13.3332, -1.605)
  line L83 (-11.8211, -1.7042) -> (-13.3134, -1.6962)
  line L84 (-10.3328, -1.7161) -> (-11.8211, -1.7042)
  line L85 (-10.0709, -2.0931) -> (-10.3328, -1.7161)
  line L86 (-9.805, -2.4702) -> (-10.0709, -2.0931)
  line L87 (-9.1938, -2.4781) -> (-9.805, -2.4702)
  line L88 (-8.5786, -2.49) -> (-9.1938, -2.4781)
  line L89 (-8.4953, -2.2955) -> (-8.5786, -2.49)
  spline S139 degree 3 poles (-7.1142, -2.5852) (-7.1142, -1.8232) (-8.1897, -1.597) (-8.4953, -2.2955) knots -1 -1 -1 -1 0 0 0 0
  spline S140 degree 3 poles (-8.023, -3.3076) (-7.5269, -3.3988) (-7.1142, -3.0694) (-7.1142, -2.5852) knots -1 -1 -1 -1 0 0 0 0
  spline S141 degree 3 poles (-8.5191, -2.8631) (-8.4596, -3.0456) (-8.2056, -3.2718) (-8.023, -3.3076) knots -1 -1 -1 -1 0 0 0 0
  line L90 (-8.5667, -2.7281) -> (-8.5191, -2.8631)
  line L91 (-9.2057, -2.7281) -> (-8.5667, -2.7281)
  spline S142 degree 3 poles (-9.8923, -2.6964) (-9.8685, -2.7122) (-9.5589, -2.7281) (-9.2057, -2.7281) knots -1 -1 -1 -1 0 0 0 0
  spline S143 degree 3 poles (-10.2019, -2.2836) (-10.055, -2.494) (-9.9121, -2.6805) (-9.8923, -2.6964) knots -1 -1 -1 -1 0 0 0 0
  line L92 (-10.4678, -1.8947) -> (-10.2019, -2.2836)
  line L93 (-11.8767, -1.8947) -> (-10.4678, -1.8947)
  spline S144 degree 3 poles (-13.2816, -1.9661) (-13.2816, -1.8987) (-13.1864, -1.8947) (-11.8767, -1.8947) knots -1 -1 -1 -1 0 0 0 0
  spline S145 degree 3 poles (-12.7816, -4.1172) (-13.0038, -3.4385) (-13.2816, -2.236) (-13.2816, -1.9661) knots -1 -1 -1 -1 0 0 0 0
  spline S146 degree 3 poles (-6.9634, -11.4713) (-9.6899, -9.8203) (-11.8052, -7.1493) (-12.7816, -4.1172) knots -1 -1 -1 -1 0 0 0 0
  spline S147 degree 3 poles (0.8273, -13.4041) (-1.8953, -13.5628) (-4.6297, -12.8842) (-6.9634, -11.4713) knots -1 -1 -1 -1 0 0 0 0
  spline S148 degree 3 poles (-9.1819, -0.9819) (-9.2375, -1.0533) (-9.3248, -1.1247) (-9.3684, -1.1406) knots -1 -1 -1 -1 0 0 0 0
  spline S149 degree 3 poles (-9.3526, -0.208) (-9.0589, -0.3588) (-8.9755, -0.7398) (-9.1819, -0.9819) knots -1 -1 -1 -1 0 0 0 0
  spline S150 degree 3 poles (-10.0669, -0.6644) (-10.0669, -0.2834) (-9.6859, -0.0373) (-9.3526, -0.208) knots -1 -1 -1 -1 0 0 0 0
  spline S151 degree 3 poles (-9.3684, -1.1406) (-9.7058, -1.2795) (-10.0669, -1.0295) (-10.0669, -0.6644) knots -1 -1 -1 -1 0 0 0 0
  spline S152 degree 3 poles (8.7846, -2.494) (8.7846, -2.6646) (8.6576, -2.8551) (8.4909, -2.9305) knots -1 -1 -1 -1 0 0 0 0
  spline S153 degree 3 poles (8.2766, -1.9741) (8.5386, -1.9741) (8.7846, -2.2281) (8.7846, -2.494) knots -1 -1 -1 -1 0 0 0 0
  spline S154 degree 3 poles (8.0464, -2.9305) (7.5583, -2.7083) (7.7329, -1.9741) (8.2766, -1.9741) knots -1 -1 -1 -1 0 0 0 0
  spline S155 degree 3 poles (8.2687, -3.0059) (8.2369, -3.0059) (8.1377, -2.9702) (8.0464, -2.9305) knots -1 -1 -1 -1 0 0 0 0
  spline S156 degree 3 poles (8.4909, -2.9305) (8.3997, -2.9702) (8.3004, -3.0059) (8.2687, -3.0059) knots -1 -1 -1 -1 0 0 0 0
  spline S157 degree 3 poles (-7.4079, -2.3432) (-7.2491, -2.5972) (-7.3523, -2.9266) (-7.6222, -3.0496) knots -1 -1 -1 -1 0 0 0 0
  spline S158 degree 3 poles (-8.3088, -2.3987) (-8.15, -2.0257) (-7.6222, -1.9899) (-7.4079, -2.3432) knots -1 -1 -1 -1 0 0 0 0
  spline S159 degree 3 poles (-8.0151, -3.0694) (-8.3008, -2.9504) (-8.4199, -2.6726) (-8.3088, -2.3987) knots -1 -1 -1 -1 0 0 0 0
  spline S160 degree 3 poles (-7.6222, -3.0496) (-7.8166, -3.1369) (-7.8524, -3.1409) (-8.0151, -3.0694) knots -1 -1 -1 -1 0 0 0 0
  spline S161 degree 3 poles (12.7216, -7.4668) (12.7018, -7.4787) (12.4041, -7.9232) (12.0589, -8.459) knots -1 -1 -1 -1 0 0 0 0
  spline S162 degree 3 poles (13.7495, -8.0899) (13.2019, -7.7367) (12.7415, -7.4549) (12.7216, -7.4668) knots -1 -1 -1 -1 0 0 0 0
  spline S163 degree 3 poles (14.7735, -8.6971) (14.7576, -8.717) (14.2933, -8.4431) (13.7495, -8.0899) knots -1 -1 -1 -1 0 0 0 0
  spline S164 degree 3 poles (15.4283, -7.6097) (15.4561, -7.6375) (14.9164, -8.5265) (14.7735, -8.6971) knots -1 -1 -1 -1 0 0 0 0
  spline S165 degree 3 poles (12.8288, -5.9309) (12.8685, -5.9388) (15.3728, -7.5581) (15.4283, -7.6097) knots -1 -1 -1 -1 0 0 0 0
  spline S166 degree 3 poles (11.785, -7.4708) (12.3367, -6.6175) (12.805, -5.9269) (12.8288, -5.9309) knots -1 -1 -1 -1 0 0 0 0
  line L94 (10.7769, -9.0186) -> (11.785, -7.4708)
  line L95 (11.0627, -9.1972) -> (10.7769, -9.0186)
  spline S167 degree 3 poles (11.3881, -9.4075) (11.3643, -9.3916) (11.2175, -9.2964) (11.0627, -9.1972) knots -1 -1 -1 -1 0 0 0 0
  spline S168 degree 3 poles (12.0589, -8.459) (11.6858, -9.0384) (11.4119, -9.4194) (11.3881, -9.4075) knots -1 -1 -1 -1 0 0 0 0
  spline S169 degree 3 poles (-10.3725, -9.5583) (-10.3924, -9.5782) (-10.9678, -9.983) (-11.6544, -10.4632) knots -1 -1 -1 -1 0 0 0 0
  spline S170 degree 3 poles (-11.837, -7.3874) (-11.3607, -8.0026) (-10.3328, -9.5187) (-10.3725, -9.5583) knots -1 -1 -1 -1 0 0 0 0
  spline S171 degree 3 poles (-12.8451, -6.4865) (-12.5236, -6.6453) (-12.1624, -6.9667) (-11.837, -7.3874) knots -1 -1 -1 -1 0 0 0 0
  spline S172 degree 3 poles (-13.365, -6.3595) (-13.1506, -6.3595) (-13.0554, -6.3833) (-12.8451, -6.4865) knots -1 -1 -1 -1 0 0 0 0
  spline S173 degree 3 poles (-13.9285, -6.5143) (-13.6666, -6.3794) (-13.5912, -6.3595) (-13.365, -6.3595) knots -1 -1 -1 -1 0 0 0 0
  spline S174 degree 3 poles (-14.8136, -7.312) (-14.6945, -7.0501) (-14.3175, -6.7088) (-13.9285, -6.5143) knots -1 -1 -1 -1 0 0 0 0
  spline S175 degree 3 poles (-14.5635, -8.9194) (-14.9128, -8.2606) (-15.0001, -7.7089) (-14.8136, -7.312) knots -1 -1 -1 -1 0 0 0 0
  spline S176 degree 3 poles (-12.9244, -11.3363) (-12.9681, -11.3443) (-14.3929, -9.2408) (-14.5635, -8.9194) knots -1 -1 -1 -1 0 0 0 0
  spline S177 degree 3 poles (-11.6544, -10.4632) (-12.341, -10.9395) (-12.9125, -11.3363) (-12.9244, -11.3363) knots -1 -1 -1 -1 0 0 0 0
  spline S178 degree 3 poles (1.5139, 15.8456) (1.5298, 14.6391) (1.5298, 14.5836) (1.4583, 14.5637) knots -1 -1 -1 -1 0 0 0 0
  spline S179 degree 3 poles (1.4821, 17.1275) (1.4901, 17.1196) (1.5059, 16.5441) (1.5139, 15.8456) knots -1 -1 -1 -1 0 0 0 0
  spline S180 degree 3 poles (0.9424, 17.1275) (1.2281, 17.1394) (1.4702, 17.1394) (1.4821, 17.1275) knots -1 -1 -1 -1 0 0 0 0
  line L96 (0.4185, 17.1037) -> (0.9424, 17.1275)
  line L97 (0.4264, 16.7426) -> (0.4185, 17.1037)
  line L98 (0.4304, 16.3814) -> (0.4264, 16.7426)
  line L99 (-0.0736, 16.3814) -> (0.4304, 16.3814)
  spline S181 degree 3 poles (-0.8753, 16.7426) (-0.7523, 16.4211) (-0.665, 16.3814) (-0.0736, 16.3814) knots -1 -1 -1 -1 0 0 0 0
  spline S182 degree 3 poles (-0.9825, 17.0243) (-0.9626, 16.9767) (-0.915, 16.8497) (-0.8753, 16.7426) knots -1 -1 -1 -1 0 0 0 0
  spline S183 degree 3 poles (-1.4905, 17.1156) (-1.0341, 17.1156) (-1.0142, 17.1117) (-0.9825, 17.0243) knots -1 -1 -1 -1 0 0 0 0
  spline S184 degree 3 poles (-1.9866, 17.0799) (-1.9746, 17.0998) (-1.7524, 17.1156) (-1.4905, 17.1156) knots -1 -1 -1 -1 0 0 0 0
  spline S185 degree 3 poles (-1.8476, 16.437) (-1.9072, 16.5441) (-2.0143, 17.0402) (-1.9866, 17.0799) knots -1 -1 -1 -1 0 0 0 0
  spline S186 degree 3 poles (-1.673, 16.2822) (-1.7524, 16.3298) (-1.8278, 16.4013) (-1.8476, 16.437) knots -1 -1 -1 -1 0 0 0 0
  line L100 (-1.5341, 16.1988) -> (-1.673, 16.2822)
  line L101 (-1.7048, 16.0718) -> (-1.5341, 16.1988)
  spline S187 degree 3 poles (-2.0104, 15.4488) (-2.0104, 15.7226) (-1.9231, 15.9052) (-1.7048, 16.0718) knots -1 -1 -1 -1 0 0 0 0
  spline S188 degree 3 poles (-1.3635, 14.6431) (-1.8278, 14.7979) (-2.0064, 15.0241) (-2.0104, 15.4488) knots -1 -1 -1 -1 0 0 0 0
  spline S189 degree 3 poles (0.1328, 14.5518) (-1.0023, 14.5598) (-1.1412, 14.5677) (-1.3635, 14.6431) knots -1 -1 -1 -1 0 0 0 0
  spline S190 degree 3 poles (1.4583, 14.5637) (1.4147, 14.5518) (0.8194, 14.5478) (0.1328, 14.5518) knots -1 -1 -1 -1 0 0 0 0
  spline S191 degree 3 poles (-3.0105, 15.9369) (-2.4866, 14.9527) (-3.0938, 14.0875) (-4.5345, 13.766) knots -1 -1 -1 -1 0 0 0 0
  spline S192 degree 3 poles (-4.8441, 16.4608) (-3.9312, 16.6949) (-3.324, 16.5203) (-3.0105, 15.9369) knots -1 -1 -1 -1 0 0 0 0
  spline S193 degree 3 poles (-6.4157, 15.0281) (-6.4157, 15.6988) (-5.864, 16.2028) (-4.8441, 16.4608) knots -1 -1 -1 -1 0 0 0 0
  spline S194 degree 3 poles (-5.7251, 13.8335) (-6.1418, 14.0438) (-6.4157, 14.524) (-6.4157, 15.0281) knots -1 -1 -1 -1 0 0 0 0
  spline S195 degree 3 poles (-4.5345, 13.766) (-4.9552, 13.6708) (-5.4711, 13.7025) (-5.7251, 13.8335) knots -1 -1 -1 -1 0 0 0 0
  spline S196 degree 3 poles (5.2882, 14.278) (5.2961, 14.27) (5.2723, 14.1351) (5.2326, 13.9803) knots -1 -1 -1 -1 0 0 0 0
  spline S197 degree 3 poles (4.8199, 14.4129) (5.0699, 14.3454) (5.2802, 14.2859) (5.2882, 14.278) knots -1 -1 -1 -1 0 0 0 0
  spline S198 degree 3 poles (4.3515, 14.5518) (4.3595, 14.5399) (4.5738, 14.4804) (4.8199, 14.4129) knots -1 -1 -1 -1 0 0 0 0
  spline S199 degree 3 poles (4.5738, 15.4924) (4.4428, 14.9844) (4.3436, 14.5598) (4.3515, 14.5518) knots -1 -1 -1 -1 0 0 0 0
  spline S200 degree 3 poles (4.8, 16.433) (4.804, 16.4251) (4.7048, 16.0004) (4.5738, 15.4924) knots -1 -1 -1 -1 0 0 0 0
  spline S201 degree 3 poles (4.2841, 16.5799) (4.5579, 16.5044) (4.7921, 16.4409) (4.8, 16.433) knots -1 -1 -1 -1 0 0 0 0
  spline S202 degree 3 poles (3.7681, 16.6473) (3.784, 16.7069) (3.8396, 16.6989) (4.2841, 16.5799) knots -1 -1 -1 -1 0 0 0 0
  spline S203 degree 3 poles (3.5221, 15.7067) (3.6491, 16.1869) (3.7562, 16.6076) (3.7681, 16.6473) knots -1 -1 -1 -1 0 0 0 0
  spline S204 degree 3 poles (3.2879, 14.8217) (3.2919, 14.8296) (3.399, 15.2265) (3.5221, 15.7067) knots -1 -1 -1 -1 0 0 0 0
  spline S205 degree 3 poles (2.8275, 14.9289) (3.0736, 14.8654) (3.28, 14.8138) (3.2879, 14.8217) knots -1 -1 -1 -1 0 0 0 0
  spline S206 degree 3 poles (2.3314, 15.0519) (2.3553, 15.0519) (2.5775, 14.9963) (2.8275, 14.9289) knots -1 -1 -1 -1 0 0 0 0
  spline S207 degree 3 poles (2.1687, 14.4685) (2.137, 14.5002) (2.2918, 15.0519) (2.3314, 15.0519) knots -1 -1 -1 -1 0 0 0 0
  spline S208 degree 3 poles (5.1175, 13.7025) (5.0619, 13.7025) (2.1886, 14.4526) (2.1687, 14.4685) knots -1 -1 -1 -1 0 0 0 0
  spline S209 degree 3 poles (5.2326, 13.9803) (5.1969, 13.8295) (5.1453, 13.7025) (5.1175, 13.7025) knots -1 -1 -1 -1 0 0 0 0
  spline S210 degree 3 poles (9.4554, 13.0874) (9.3045, 12.6786) (8.9751, 12.3452) (8.6378, 12.2499) knots -1 -1 -1 -1 0 0 0 0
  spline S211 degree 3 poles (8.2885, 14.9924) (9.3045, 14.4764) (9.7213, 13.7978) (9.4554, 13.0874) knots -1 -1 -1 -1 0 0 0 0
  spline S212 degree 3 poles (7.2686, 15.29) (7.5821, 15.29) (7.8718, 15.2067) (8.2885, 14.9924) knots -1 -1 -1 -1 0 0 0 0
  spline S213 degree 3 poles (6.5264, 15.036) (6.6534, 15.1709) (6.9987, 15.29) (7.2686, 15.29) knots -1 -1 -1 -1 0 0 0 0
  line L102 (6.4351, 14.9408) -> (6.5264, 15.036)
  line L103 (6.709, 14.782) -> (6.4351, 14.9408)
  spline S214 degree 3 poles (7.4749, 14.4169) (7.4154, 14.3812) (7.344, 14.4129) (6.709, 14.782) knots -1 -1 -1 -1 0 0 0 0
  spline S215 degree 3 poles (8.0663, 14.3534) (7.852, 14.4605) (7.5861, 14.4883) (7.4749, 14.4169) knots -1 -1 -1 -1 0 0 0 0
  spline S216 degree 3 poles (8.4513, 13.4525) (8.6021, 13.8097) (8.4513, 14.1589) (8.0663, 14.3534) knots -1 -1 -1 -1 0 0 0 0
  spline S217 degree 3 poles (7.975, 13.0437) (8.1417, 13.0754) (8.3798, 13.2779) (8.4513, 13.4525) knots -1 -1 -1 -1 0 0 0 0
  spline S218 degree 3 poles (7.0662, 13.5954) (7.1733, 13.2779) (7.6575, 12.9842) (7.975, 13.0437) knots -1 -1 -1 -1 0 0 0 0
  spline S219 degree 3 poles (6.5423, 14.0319) (6.9828, 13.7779) (7.0146, 13.7501) (7.0662, 13.5954) knots -1 -1 -1 -1 0 0 0 0
  spline S220 degree 3 poles (6.0502, 14.274) (6.0621, 14.2899) (6.2843, 14.1788) (6.5423, 14.0319) knots -1 -1 -1 -1 0 0 0 0
  spline S221 degree 3 poles (6.0303, 13.9843) (6.0264, 14.1311) (6.0383, 14.2621) (6.0502, 14.274) knots -1 -1 -1 -1 0 0 0 0
  spline S222 degree 3 poles (6.5145, 13.0199) (6.1653, 13.3493) (6.0303, 13.6152) (6.0303, 13.9843) knots -1 -1 -1 -1 0 0 0 0
  spline S223 degree 3 poles (8.6378, 12.2499) (8.0742, 12.0912) (7.1495, 12.4246) (6.5145, 13.0199) knots -1 -1 -1 -1 0 0 0 0
  line L104 (-8.8446, 11.5316) -> (-9.2851, 11.23)
  line L105 (-9.3406, 12.2658) -> (-8.8446, 11.5316)
  spline S224 degree 3 poles (-9.7653, 12.9762) (-9.8129, 12.9881) (-9.6661, 12.7421) (-9.3406, 12.2658) knots -1 -1 -1 -1 0 0 0 0
  spline S225 degree 3 poles (-7.6341, 12.3928) (-7.6777, 12.3928) (-9.2692, 12.8254) (-9.7653, 12.9762) knots -1 -1 -1 -1 0 0 0 0
  spline S226 degree 3 poles (-6.5943, 13.1112) (-6.5943, 13.0556) (-7.5547, 12.3928) (-7.6341, 12.3928) knots -1 -1 -1 -1 0 0 0 0
  spline S227 degree 3 poles (-8.0111, 15.2106) (-7.9714, 15.2067) (-6.5943, 13.1667) (-6.5943, 13.1112) knots -1 -1 -1 -1 0 0 0 0
  spline S228 degree 3 poles (-8.8525, 14.6034) (-8.8565, 14.6471) (-8.0706, 15.2106) (-8.0111, 15.2106) knots -1 -1 -1 -1 0 0 0 0
  spline S229 degree 3 poles (-8.3842, 13.8811) (-8.6382, 14.2542) (-8.8485, 14.5756) (-8.8525, 14.6034) knots -1 -1 -1 -1 0 0 0 0
  spline S230 degree 3 poles (-7.9595, 13.1945) (-7.9397, 13.2024) (-8.1302, 13.512) (-8.3842, 13.8811) knots -1 -1 -1 -1 0 0 0 0
  spline S231 degree 3 poles (-9.0589, 13.4842) (-8.4755, 13.3175) (-7.9794, 13.1866) (-7.9595, 13.1945) knots -1 -1 -1 -1 0 0 0 0
  line L106 (-10.1225, 13.7858) -> (-9.0589, 13.4842)
  line L107 (-10.6345, 13.4366) -> (-10.1225, 13.7858)
  spline S232 degree 3 poles (-11.1583, 13.0675) (-11.1504, 13.0794) (-10.9123, 13.2461) (-10.6345, 13.4366) knots -1 -1 -1 -1 0 0 0 0
  spline S233 degree 3 poles (-9.7851, 11.0157) (-10.2416, 11.6626) (-11.1702, 13.0516) (-11.1583, 13.0675) knots -1 -1 -1 -1 0 0 0 0
  spline S234 degree 3 poles (-9.2851, 11.23) (-9.7256, 10.9283) (-9.7256, 10.9283) (-9.7851, 11.0157) knots -1 -1 -1 -1 0 0 0 0
  spline S235 degree 3 poles (-10.2971, 10.2338) (-10.3011, 10.2179) (-10.4638, 10.0354) (-10.6503, 9.833) knots -1 -1 -1 -1 0 0 0 0
  spline S236 degree 3 poles (-11.0591, 10.9799) (-10.6345, 10.591) (-10.2892, 10.2537) (-10.2971, 10.2338) knots -1 -1 -1 -1 0 0 0 0
  spline S237 degree 3 poles (-11.9997, 11.8491) (-11.9084, 11.7618) (-11.4838, 11.3728) (-11.0591, 10.9799) knots -1 -1 -1 -1 0 0 0 0
  line L108 (-12.1624, 12.0078) -> (-11.9997, 11.8491)
  line L109 (-12.4006, 11.7538) -> (-12.1624, 12.0078)
  spline S238 degree 3 poles (-12.7617, 11.357) (-12.6903, 11.4363) (-12.5276, 11.6149) (-12.4006, 11.7538) knots -1 -1 -1 -1 0 0 0 0
  line L110 (-12.8847, 11.2101) -> (-12.7617, 11.357)
  line L111 (-11.9402, 10.337) -> (-12.8847, 11.2101)
  line L112 (-10.9916, 9.4639) -> (-11.9402, 10.337)
  line L113 (-10.6503, 9.833) -> (-10.9916, 9.4639)
  line L114 (13.1701, 10.9919) -> (12.2573, 10.1068)
  line L115 (12.0787, 12.111) -> (13.1701, 10.9919)
  line L116 (10.9913, 13.2302) -> (12.0787, 12.111)
  line L117 (10.7809, 13.0199) -> (10.9913, 13.2302)
  spline S239 degree 3 poles (10.5706, 12.7738) (10.5706, 12.7976) (10.6658, 12.9048) (10.7809, 13.0199) knots -1 -1 -1 -1 0 0 0 0
  spline S240 degree 3 poles (11.2651, 12.0396) (10.8841, 12.4246) (10.5706, 12.754) (10.5706, 12.7738) knots -1 -1 -1 -1 0 0 0 0
  line L118 (11.9596, 11.3371) -> (11.2651, 12.0396)
  line L119 (11.8088, 11.1903) -> (11.9596, 11.3371)
  line L120 (11.662, 11.0434) -> (11.8088, 11.1903)
  line L121 (10.5309, 12.1745) -> (11.662, 11.0434)
  line L122 (10.3642, 12.0039) -> (10.5309, 12.1745)
  line L123 (10.1935, 11.8372) -> (10.3642, 12.0039)
  line L124 (10.7611, 11.2697) -> (10.1935, 11.8372)
  line L125 (11.3246, 10.7021) -> (10.7611, 11.2697)
  line L126 (11.0151, 10.4005) -> (11.3246, 10.7021)
  line L127 (10.3721, 11.0593) -> (11.0151, 10.4005)
  spline S241 degree 3 poles (9.6816, 11.7181) (9.7054, 11.7181) (10.0149, 11.4205) (10.3721, 11.0593) knots -1 -1 -1 -1 0 0 0 0
  spline S242 degree 3 poles (9.4395, 11.5197) (9.5466, 11.6308) (9.6538, 11.7181) (9.6816, 11.7181) knots -1 -1 -1 -1 0 0 0 0
  line L128 (9.245, 11.3213) -> (9.4395, 11.5197)
  line L129 (9.3998, 11.1546) -> (9.245, 11.3213)
  spline S243 degree 3 poles (11.3246, 9.2178) (11.3048, 9.2178) (9.6895, 10.841) (9.3998, 11.1546) knots -1 -1 -1 -1 0 0 0 0
  spline S244 degree 3 poles (12.2573, 10.1068) (11.7533, 9.6187) (11.3365, 9.2178) (11.3246, 9.2178) knots -1 -1 -1 -1 0 0 0 0
  spline S245 degree 3 poles (-12.8133, 6.8167) (-13.0832, 6.527) (-13.2578, 6.404) (-13.5197, 6.3325) knots -1 -1 -1 -1 0 0 0 0
  spline S246 degree 3 poles (-12.1188, 7.9835) (-12.2696, 7.547) (-12.5156, 7.1342) (-12.8133, 6.8167) knots -1 -1 -1 -1 0 0 0 0
  spline S247 degree 3 poles (-12.0196, 8.6185) (-12.0037, 8.3645) (-12.0196, 8.2733) (-12.1188, 7.9835) knots -1 -1 -1 -1 0 0 0 0
  spline S248 degree 3 poles (-12.1227, 9.0789) (-12.0672, 8.9757) (-12.0315, 8.817) (-12.0196, 8.6185) knots -1 -1 -1 -1 0 0 0 0
  spline S249 degree 3 poles (-13.1943, 9.8012) (-12.7736, 9.7496) (-12.3053, 9.4361) (-12.1227, 9.0789) knots -1 -1 -1 -1 0 0 0 0
  spline S250 degree 3 poles (-14.7223, 8.7217) (-14.2778, 9.4758) (-13.7261, 9.8647) (-13.1943, 9.8012) knots -1 -1 -1 -1 0 0 0 0
  spline S251 degree 3 poles (-14.8771, 6.8405) (-15.2263, 7.2573) (-15.1668, 7.9637) (-14.7223, 8.7217) knots -1 -1 -1 -1 0 0 0 0
  line L130 (-14.7699, 6.7096) -> (-14.8771, 6.8405)
  line L131 (-14.4841, 7.1977) -> (-14.7699, 6.7096)
  spline S252 degree 3 poles (-14.2381, 7.7772) (-14.2063, 7.6978) (-14.246, 7.6065) (-14.4841, 7.1977) knots -1 -1 -1 -1 0 0 0 0
  spline S253 degree 3 poles (-13.7896, 8.7257) (-14.119, 8.5511) (-14.3492, 8.0708) (-14.2381, 7.7772) knots -1 -1 -1 -1 0 0 0 0
  spline S254 degree 3 poles (-12.9403, 8.4399) (-13.111, 8.7336) (-13.5158, 8.8686) (-13.7896, 8.7257) knots -1 -1 -1 -1 0 0 0 0
  spline S255 degree 3 poles (-12.9403, 7.8089) (-12.8212, 8.0629) (-12.8212, 8.2375) (-12.9403, 8.4399) knots -1 -1 -1 -1 0 0 0 0
  spline S256 degree 3 poles (-13.4245, 7.3327) (-13.2221, 7.4041) (-13.0554, 7.5668) (-12.9403, 7.8089) knots -1 -1 -1 -1 0 0 0 0
  spline S257 degree 3 poles (-13.8531, 6.8207) (-13.6071, 7.2334) (-13.5634, 7.289) (-13.4245, 7.3327) knots -1 -1 -1 -1 0 0 0 0
  spline S258 degree 3 poles (-14.1071, 6.3365) (-14.1151, 6.3484) (-14.0039, 6.5667) (-13.8531, 6.8207) knots -1 -1 -1 -1 0 0 0 0
  spline S259 degree 3 poles (-13.5197, 6.3325) (-13.6825, 6.2849) (-14.0595, 6.2889) (-14.1071, 6.3365) knots -1 -1 -1 -1 0 0 0 0
  spline S260 degree 3 poles (1.6726, -13.9597) (1.6647, -13.9756) (1.1686, -14.6542) (0.5693, -15.4638) knots -1 -1 -1 -1 0 0 0 0
  spline S261 degree 3 poles (1.3353, -13.9041) (1.5258, -13.92) (1.6766, -13.9438) (1.6726, -13.9597) knots -1 -1 -1 -1 0 0 0 0
  spline S262 degree 3 poles (0.6844, -13.8565) (0.8511, -13.8684) (1.1448, -13.8922) (1.3353, -13.9041) knots -1 -1 -1 -1 0 0 0 0
  line L132 (0.3788, -13.8327) -> (0.6844, -13.8565)
  line L133 (0.2161, -14.0748) -> (0.3788, -13.8327)
  spline S263 degree 3 poles (-1.1174, -14.2573) (0.1129, -14.3486) (0.0216, -14.3605) (0.2161, -14.0748) knots -1 -1 -1 -1 0 0 0 0
  spline S264 degree 3 poles (-1.9548, -14.1978) (-1.931, -14.1978) (-1.554, -14.2256) (-1.1174, -14.2573) knots -1 -1 -1 -1 0 0 0 0
  spline S265 degree 3 poles (-2.1255, -13.9279) (-2.054, -14.0748) (-1.9786, -14.1978) (-1.9548, -14.1978) knots -1 -1 -1 -1 0 0 0 0
  line L134 (-2.2485, -13.6541) -> (-2.1255, -13.9279)
  line L135 (-2.8914, -13.6104) -> (-2.2485, -13.6541)
  spline S266 degree 3 poles (-3.5463, -13.5787) (-3.5383, -13.5707) (-3.2446, -13.5827) (-2.8914, -13.6104) knots -1 -1 -1 -1 0 0 0 0
  spline S267 degree 3 poles (-2.6811, -15.2098) (-3.1653, -14.3208) (-3.5582, -13.5866) (-3.5463, -13.5787) knots -1 -1 -1 -1 0 0 0 0
  spline S268 degree 3 poles (-1.7167, -16.8569) (-1.7722, -16.8331) (-2.0659, -16.333) (-2.6811, -15.2098) knots -1 -1 -1 -1 0 0 0 0
  spline S269 degree 3 poles (-1.0777, -16.9164) (-1.3793, -16.9005) (-1.6691, -16.8727) (-1.7167, -16.8569) knots -1 -1 -1 -1 0 0 0 0
  line L136 (-0.5221, -16.9402) -> (-1.0777, -16.9164)
  line L137 (0.5693, -15.4638) -> (-0.5221, -16.9402)
  spline S270 degree 3 poles (7.721, -15.2575) (7.6853, -15.2733) (6.9312, -15.5591) (6.0462, -15.8885) knots -1 -1 -1 -1 0 0 0 0
  spline S271 degree 3 poles (7.6654, -14.8844) (7.7805, -15.2019) (7.7845, -15.2336) (7.721, -15.2575) knots -1 -1 -1 -1 0 0 0 0
  spline S272 degree 3 poles (7.5345, -14.5272) (7.5384, -14.5312) (7.598, -14.6939) (7.6654, -14.8844) knots -1 -1 -1 -1 0 0 0 0
  spline S273 degree 3 poles (6.5621, -14.8725) (7.0939, -14.678) (7.5305, -14.5193) (7.5345, -14.5272) knots -1 -1 -1 -1 0 0 0 0
  spline S274 degree 3 poles (5.5819, -15.2138) (5.5898, -15.2257) (6.0343, -15.0709) (6.5621, -14.8725) knots -1 -1 -1 -1 0 0 0 0
  spline S275 degree 3 poles (6.2605, -14.0906) (5.8755, -14.6979) (5.5699, -15.2059) (5.5819, -15.2138) knots -1 -1 -1 -1 0 0 0 0
  line L138 (6.955, -12.9834) -> (6.2605, -14.0906)
  line L139 (6.8201, -12.6262) -> (6.955, -12.9834)
  spline S276 degree 3 poles (6.6336, -12.2849) (6.6693, -12.2769) (6.7368, -12.4) (6.8201, -12.6262) knots -1 -1 -1 -1 0 0 0 0
  spline S277 degree 3 poles (3.2681, -13.5787) (3.2681, -13.543) (6.3915, -12.3444) (6.6336, -12.2849) knots -1 -1 -1 -1 0 0 0 0
  spline S278 degree 3 poles (3.53, -14.2256) (3.4943, -14.2137) (3.2681, -13.6581) (3.2681, -13.5787) knots -1 -1 -1 -1 0 0 0 0
  spline S279 degree 3 poles (4.5182, -13.8843) (3.9944, -14.0787) (3.5499, -14.2335) (3.53, -14.2256) knots -1 -1 -1 -1 0 0 0 0
  spline S280 degree 3 poles (5.4826, -13.539) (5.4747, -13.535) (5.0421, -13.6898) (4.5182, -13.8843) knots -1 -1 -1 -1 0 0 0 0
  spline S281 degree 3 poles (4.796, -14.6542) (5.181, -14.047) (5.4866, -13.5469) (5.4826, -13.539) knots -1 -1 -1 -1 0 0 0 0
  spline S282 degree 3 poles (4.1015, -15.8091) (4.1015, -15.7813) (4.415, -15.2654) (4.796, -14.6542) knots -1 -1 -1 -1 0 0 0 0
  spline S283 degree 3 poles (4.3912, -16.4957) (4.3476, -16.4997) (4.1015, -15.9163) (4.1015, -15.8091) knots -1 -1 -1 -1 0 0 0 0
  spline S284 degree 3 poles (6.0462, -15.8885) (5.1612, -16.2219) (4.419, -16.4957) (4.3912, -16.4957) knots -1 -1 -1 -1 0 0 0 0
  spline S285 degree 3 poles (-5.8878, -14.1621) (-6.2688, -14.8249) (-6.626, -15.444) (-6.6776, -15.5392) knots -1 -1 -1 -1 0 0 0 0
  line L140 (-5.1933, -12.9516) -> (-5.8878, -14.1621)
  line L141 (-5.7331, -12.6381) -> (-5.1933, -12.9516)
  spline S286 degree 3 poles (-6.3085, -12.3206) (-6.2926, -12.3246) (-6.0307, -12.4674) (-5.7331, -12.6381) knots -1 -1 -1 -1 0 0 0 0
  spline S287 degree 3 poles (-6.5625, -12.6897) (-6.4395, -12.4833) (-6.3284, -12.3166) (-6.3085, -12.3206) knots -1 -1 -1 -1 0 0 0 0
  spline S288 degree 3 poles (-6.7927, -13.0826) (-6.7848, -13.0747) (-6.6816, -12.8961) (-6.5625, -12.6897) knots -1 -1 -1 -1 0 0 0 0
  spline S289 degree 3 poles (-7.8127, -12.4635) (-7.7412, -12.5468) (-6.8165, -13.1024) (-6.7927, -13.0826) knots -1 -1 -1 -1 0 0 0 0
  spline S290 degree 3 poles (-7.9436, -12.2412) (-7.9079, -12.3206) (-7.8524, -12.4238) (-7.8127, -12.4635) knots -1 -1 -1 -1 0 0 0 0
  spline S291 degree 3 poles (-7.9436, -11.8324) (-7.9992, -12.0666) (-7.9992, -12.1063) (-7.9436, -12.2412) knots -1 -1 -1 -1 0 0 0 0
  spline S292 degree 3 poles (-8.4159, -11.0982) (-7.8206, -11.4356) (-7.8444, -11.3998) (-7.9436, -11.8324) knots -1 -1 -1 -1 0 0 0 0
  line L142 (-8.9438, -10.7966) -> (-8.4159, -11.0982)
  line L143 (-9.047, -11.122) -> (-8.9438, -10.7966)
  spline S293 degree 3 poles (-9.0747, -11.8959) (-9.1819, -11.6896) (-9.174, -11.507) (-9.047, -11.122) knots -1 -1 -1 -1 0 0 0 0
  spline S294 degree 3 poles (-9.0946, -12.0666) (-8.9755, -12.0864) (-8.9755, -12.0904) (-9.0747, -11.8959) knots -1 -1 -1 -1 0 0 0 0
  spline S295 degree 3 poles (-9.7455, -12.2769) (-9.5748, -12.1341) (-9.2652, -12.0309) (-9.0946, -12.0666) knots -1 -1 -1 -1 0 0 0 0
  spline S296 degree 3 poles (-10.1225, -13.0588) (-10.1185, -12.7929) (-9.9558, -12.4595) (-9.7455, -12.2769) knots -1 -1 -1 -1 0 0 0 0
  spline S297 degree 3 poles (-9.7296, -13.8525) (-10.0034, -13.5787) (-10.1225, -13.3326) (-10.1225, -13.0588) knots -1 -1 -1 -1 0 0 0 0
  spline S298 degree 3 poles (-7.8841, -15.0709) (-9.0827, -14.3804) (-9.428, -14.1542) (-9.7296, -13.8525) knots -1 -1 -1 -1 0 0 0 0
  spline S299 degree 3 poles (-6.8046, -15.6901) (-6.8205, -15.6821) (-7.3047, -15.4043) (-7.8841, -15.0709) knots -1 -1 -1 -1 0 0 0 0
  spline S300 degree 3 poles (-6.6776, -15.5392) (-6.7332, -15.6305) (-6.7887, -15.702) (-6.8046, -15.6901) knots -1 -1 -1 -1 0 0 0 0
  spline S301 degree 3 poles (11.2889, -12.7135) (11.3127, -12.7413) (11.1421, -12.9) (10.8166, -13.158) knots -1 -1 -1 -1 0 0 0 0
  spline S302 degree 3 poles (10.2967, -11.4673) (10.8246, -12.1301) (11.273, -12.6897) (11.2889, -12.7135) knots -1 -1 -1 -1 0 0 0 0
  line L144 (9.3363, -10.2687) -> (10.2967, -11.4673)